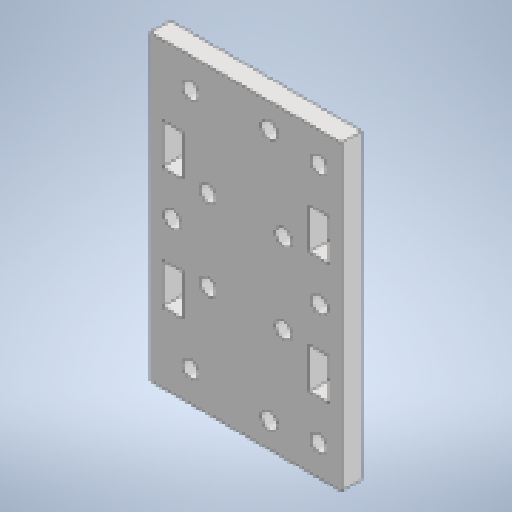
# Autodesk Inventor part: пол_каретки
Saved by Autodesk Inventor 2023.1 (Build 271208000, 208)
## iProperties
Created: 2026-01-30
Part Number: пол_каретки
Material: Типовые
Document SubType Name: Modeling
Designer: DELL
Density: 1 g/cm^3
Appearance: По умолчанию
Author: DELL
Autodesk Inventor part; units mm, degrees
ref_plane "YZ Plane" through (0, 0, 0) normal (1, 0, 0) x (0, 1, 0)
ref_plane "XZ Plane" through (0, 0, 0) normal (0, 1, 0) x (-1, 0, 0)
ref_plane "XY Plane" through (0, 0, 0) normal (0, 0, 1) x (1, 0, 0)
sketch "Эскиз1" plane through (0, 0, 0) normal (0, 0, 1) x (1, 0, 0)
  circle A0 centre (-7.5, -6.95) radius 1.5 construction
  circle A1 centre (7.5, -6.95) radius 1.5 construction
  circle A2 centre (-7.5, -22.95) radius 1.5 construction
  circle A3 centre (7.5, -22.95) radius 1.5 construction
  circle A4 centre (-7.5, -6.95) radius 1.6
  circle A5 centre (7.5, -6.95) radius 1.6
  circle A6 centre (7.5, -22.95) radius 1.6
  circle A7 centre (-7.5, -22.95) radius 1.6
  line L0 (-7.5, -6.95) -> (7.5, -22.95) construction
  line L1 (-19, 15.05) -> (19, 15.05)
  line L2 (19, 15.05) -> (19, -44.95)
  line L3 (19, -44.95) -> (-19, -44.95)
  line L4 (-19, -44.95) -> (-19, 15.05)
  line L5 (-19, 15.05) -> (19, -44.95) construction
  line L6 (19, 15.05) -> (-19, -44.95) construction
  point P0 (0, 0)
  point P1 (0, -14.95)
  dimension "d0" = 3.2
  dimension "d1" = 3.2
  dimension "d2" = 3.2
  dimension "d3" = 3.2
  dimension "d4" = 38
  dimension "d5" = 60
  constraints: 14 end point, 4 centre point, 4 coincident, 3 midpoint, 2 parallel, 1 horizontal, 1 perpendicular
  measures "d0" diameter of A4
  measures "d1" diameter of A5
  measures "d2" diameter of A6
  measures "d3" diameter of A7
  measures "d4" distance of L2.end L3.end
  measures "d5" distance of L1.end L2.end
extrude "Выдавливание1" add sketch "Эскиз1" along normal blind 4
sketch "Эскиз2" plane through (0, 0, 4) normal (0, 0, 1) x (1, 0, 0)
  circle A0 centre (-7.5, -22.95) radius 1.6 construction
  circle A1 centre (7.5, -6.95) radius 1.6 construction
  circle A2 centre (7.5, -6.95) radius 1.6 construction
  line L0 (-7.5, -22.95) -> (7.5, -6.95) construction
  line L1 (16.6, -30.95) -> (-16.6, -30.95) construction
  line L2 (-16.6, -30.95) -> (-16.6, 1.05) construction
  line L3 (-16.6, 1.05) -> (16.6, 1.05) construction
  line L4 (16.6, 1.05) -> (16.6, -30.95) construction
  line L5 (16.6, -30.95) -> (-16.6, 1.05) construction
  line L6 (-16.6, -30.95) -> (16.6, 1.05) construction
  line L7 (-16.6, -30.95) -> (-12.6, -30.95)
  line L8 (-12.6, -30.95) -> (-12.6, -22.95)
  line L9 (-12.6, -22.95) -> (-16.6, -22.95)
  line L10 (-16.6, -22.95) -> (-16.6, -30.95)
  line L11 (-16.6, 1.05) -> (-12.6, 1.05)
  line L12 (-12.6, 1.05) -> (-12.6, -6.95)
  line L13 (-12.6, -6.95) -> (-16.6, -6.95)
  line L14 (-16.6, -6.95) -> (-16.6, 1.05)
  line L15 (16.6, -30.95) -> (12.6, -30.95)
  line L16 (12.6, -30.95) -> (12.6, -22.95)
  line L17 (12.6, -22.95) -> (16.6, -22.95)
  line L18 (16.6, -22.95) -> (16.6, -30.95)
  line L19 (16.6, 1.05) -> (12.6, 1.05)
  line L20 (12.6, 1.05) -> (12.6, -6.95)
  line L21 (12.6, -6.95) -> (16.6, -6.95)
  line L22 (16.6, -6.95) -> (16.6, 1.05)
  point P0 (0, -14.95)
  dimension "d41" = 33.2
  dimension "d42" = 32
  dimension "d43" = 4
  dimension "d44" = 8
  dimension "d45" = 4
  dimension "d46" = 8
  dimension "d47" = 4
  dimension "d48" = 4
  dimension "d49" = 8
  dimension "d50" = 8
  constraints: 46 end point, 10 parallel, 5 horizontal, 5 perpendicular, 3 midpoint
  measures "d41" distance of L2.end L3.end
  measures "d42" distance of L1.end L2.end
  measures "d43" distance of L9.end L8.end
  measures "d44" distance of L8.end L7.end
  measures "d45" distance of L12.end L13.end
  measures "d46" distance of L11.end L12.end
  measures "d47" distance of L16.end L17.end
  measures "d48" distance of L21.end L20.end
  measures "d49" distance of L20.end L19.end
  measures "d50" distance of L15.end L16.end
extrude "Выдавливание2" cut sketch "Эскиз2" against normal blind 4
sketch "Эскиз3" plane through (0, 0, 4) normal (0, 0, 1) x (1, 0, 0)
  line L0 (12.6, -22.95) -> (16.6, -22.95) construction
  line L1 (16.6, -6.95) -> (12.6, -6.95) construction
  line L2 (14.6, -22.95) -> (14.6, -6.95) construction
  circle A0 centre (14.6, -14.95) radius 1.65
  line L3 (-19, -44.95) -> (19, -44.95) projected
  line L4 (0, -44.95) -> (0, 15.05) construction
  line L5 (19, 15.05) -> (-19, 15.05) projected
  circle A1 centre (-14.6, -14.95) radius 1.65
  point P0 (0, 0)
  dimension "d18" = 3.3
  constraints: 8 end point, 3 midpoint, 2 centre point, 1 symmetric about line, 1 other
  measures "d18" diameter of A0
extrude "Выдавливание3" cut sketch "Эскиз3" against normal blind 10
sketch "Эскиз4" plane through (0, 0, 4) normal (0, 0, 1) x (1, 0, 0)
  line L0 (19, -44.95) -> (19, 15.05) projected
  line L1 (19, -14.95) -> (-2.8531, -14.95) construction
  line L2 (4.6, -39.95) -> (4.6, 10.05) construction
  circle A0 centre (4.6, -39.95) radius 1.6
  circle A1 centre (4.6, 10.05) radius 1.6
  point P0 (0, 0)
  point P1 (4.6, -14.95)
  dimension "d22" = 50
  dimension "d24" = 3.2
  dimension "d25" = 3.2
  constraints: 4 end point, 2 centre point, 2 coincident, 2 midpoint, 1 horizontal, 1 point on line, 1 vertical
  measures "d22" distance of L2.start L2.end
  measures "d24" diameter of A0
  measures "d25" diameter of A1
extrude "Выдавливание4" cut sketch "Эскиз4" against normal blind 10
sketch "Эскиз5" plane through (0, 0, 4) normal (0, 0, 1) x (1, 0, 0)
  line L0 (16.6, -30.95) -> (12.6, -30.95) construction
  line L1 (16.6, 1.05) -> (12.6, 1.05) construction
  line L2 (-12.6, 1.05) -> (-16.6, 1.05) construction
  line L3 (-12.6, -30.95) -> (-16.6, -30.95) construction
  circle A0 centre (14.5, -38.95) radius 1.6
  line L4 (19, -44.95) -> (19, 15.05) projected
  line L5 (19, -14.95) -> (-19, -14.95) construction
  line L6 (-19, 15.05) -> (-19, -44.95) projected
  line L7 (19, 15.05) -> (-19, 15.05) projected
  line L8 (0, 15.05) -> (0, -44.95) construction
  line L9 (-19, -44.95) -> (19, -44.95) projected
  circle A1 centre (14.5, 9.05) radius 1.6
  line L10 (0, -44.95) -> (0, 15.05) construction
  line L11 (-16.6, -30.95) -> (-12.6, -30.95) construction
  line L12 (-16.6, 1.05) -> (-12.6, 1.05) construction
  circle A2 centre (-11, -38.95) radius 1.6
  circle A3 centre (-11, 9.05) radius 1.6
  point P0 (0, 0)
  dimension "d28" = 3.2
  dimension "d33" = 3.2
  dimension "d34" = 3.2
  dimension "d35" = 6
  dimension "d36" = 6
  dimension "d37" = 8
  dimension "d38" = 8
  dimension "d39" = 6
  dimension "d40" = 4.5
  constraints: 10 end point, 4 centre point, 4 midpoint, 3 symmetric about line, 1 other
  measures "d28" diameter of A0
  measures "d33" diameter of A2
  measures "d34" diameter of A3
  measures "d35" distance from line of L7 A3.centre
  measures "d36" distance from line of L9 A2.centre
  measures "d37" distance from line of L6 A2.centre
  measures "d38" distance from line of L6 A3.centre
  measures "d39" distance from line of L9 A0.centre
  measures "d40" distance from line of L4 A0.centre
extrude "Выдавливание5" cut sketch "Эскиз5" against normal blind 10 contours A0 | A1 | A2 | A3
